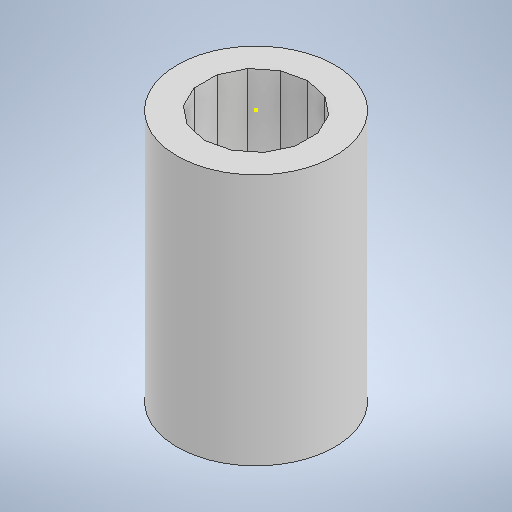
# Autodesk Inventor part: spool_motor
Saved by Autodesk Inventor 2025.2 (Build 292293000, 293)
## iProperties
Created: 2024-12-25
Part Number: spool_motor
Material: Ogólny
Document SubType Name: Modeling
Designer: Mos
Density: 1 g/cm^3
Appearance: Domyślna
Author: Mos
Autodesk Inventor part; units mm, degrees
ref_plane "YZ Plane" through (0, 0, 0) normal (1, 0, 0) x (0, 1, 0)
ref_plane "XZ Plane" through (0, 0, 0) normal (0, 1, 0) x (-1, 0, 0)
ref_plane "XY Plane" through (0, 0, 0) normal (0, 0, 1) x (1, 0, 0)
sketch "Szkic1" plane through (0, 0, 0) normal (0, 1, 0) x (-1, 0, 0)
  circle A0 centre (0, 0) radius 9.915
  constraints: 1 centre point, 1 coincident
extrude "Wyciągnięcie proste1" add sketch "Szkic1" along normal blind 31.7
sketch "Szkic2" plane through (0, 31.7, 0) normal (0, 1, 0) x (1, 0, 0)
  point P0 (0, 0)
sketch "Szkic3" plane through (0, 31.7, 0) normal (0, 1, 0) x (1, 0, 0)
  point P0 (0, 0)
sketch "Szkic4" plane through (0, 31.7, 0) normal (0, 1, 0) x (1, 0, 0)
  line L0 (6.337, -1.4464) -> (5.0819, -4.0527)
  line L1 (5.0819, -4.0527) -> (2.8202, -5.8563)
  line L2 (2.8202, -5.8563) -> (0, -6.5)
  line L3 (0, -6.5) -> (-2.8202, -5.8563)
  line L4 (-2.8202, -5.8563) -> (-5.0819, -4.0527)
  line L5 (-5.0819, -4.0527) -> (-6.337, -1.4464)
  line L6 (-6.337, -1.4464) -> (-6.337, 1.4464)
  line L7 (-6.337, 1.4464) -> (-5.0819, 4.0527)
  line L8 (-5.0819, 4.0527) -> (-2.8202, 5.8563)
  line L9 (-2.8202, 5.8563) -> (0, 6.5)
  line L10 (0, 6.5) -> (2.8202, 5.8563)
  line L11 (2.8202, 5.8563) -> (5.0819, 4.0527)
  line L12 (5.0819, 4.0527) -> (6.337, 1.4464)
  line L13 (6.337, 1.4464) -> (6.337, -1.4464)
  point P0 (0, 0)
  point P1 (0, 0)
  dimension "d2" = 6.5
  constraints: 28 end point, 1 coincident, 29 other
  measures "d2" distance of L12.end point (0, 0)
extrude "Wyciągnięcie proste2" cut sketch "Szkic4" against normal blind 40
